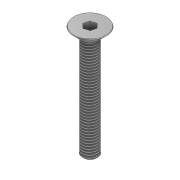
# Autodesk Inventor part: Tornillo Allen cabeza fresada M3x20mm
Saved by Autodesk Inventor 2020.3 (Build 243373000, 373)
## iProperties
Created: 2020-05-08
Part Number: Tornillo Allen cabeza fresada M3x20mm
Material: Generic
Document SubType Name: Modeling
Designer: Dante
Density: 1 g/cm^3
Appearance: Rubber - Black - Version 1.1
Mass: 0.242439 g
Surface Area: 2.80465 cm^2
Volume: 0.242439 cm^3
Author: Dante
Autodesk Inventor part; units mm, degrees
ref_plane "YZ Plane" through (0, 0, 0) normal (1, 0, 0) x (0, 1, 0)
ref_plane "XZ Plane" through (0, 0, 0) normal (0, 1, 0) x (-1, 0, 0)
ref_plane "XY Plane" through (0, 0, 0) normal (0, 0, 1) x (1, 0, 0)
sketch "Sketch1" plane through (0, 0, 0) normal (0, 0, 1) x (1, 0, 0)
  line L0 (-13.7828, -22.52) -> (-10.4228, -22.52)
  line L1 (-10.4228, -22.52) -> (-10.4228, -29.38)
  line L2 (-10.4228, -29.38) -> (-10.4228, -44.38)
  line L3 (-10.4228, -44.38) -> (-11.9228, -44.38)
  line L4 (-11.9228, -44.38) -> (-11.9228, -24.38)
  line L5 (-11.9228, -24.38) -> (-13.7828, -22.52)
  point P0 (0, 0)
  dimension "d3" = 1.5
  dimension "d15" = 1.86
  dimension "d16" = 3.36
  dimension "d23" = 20
  dimension "d24" = 21.86
  constraints: 12 end point, 2 perpendicular, 2 vertical
  measures "d3" distance of L2.end L3.end
  measures "d15" distance from line of L0 L4.end
  measures "d16" distance of L0.end L0.start
  measures "d23" distance of L3.end L4.end
  measures "d24" distance from line of L2.end L0
revolve "Revolution1" add sketch "Sketch1" angle 360 about axis through (-10.4228, -29.38, 0) along (0, -1, 0)
chamfer "Chamfer2" distance 0.2 angle 45 1 edges at (-8.9228, -44.38, 0)
chamfer "Chaflán3" distance 0.2 angle 45 1 edges at (-7.0628, -22.52, 0)
sketch "Boceto2" plane through (-10.4228, -22.52, 0) normal (0, 1, 0) x (1, 0, 0)
  line L0 (-0.8371, 0.7954) -> (0.2703, 1.1226)
  line L1 (0.2703, 1.1226) -> (1.1074, 0.3272)
  line L2 (1.1074, 0.3272) -> (0.8371, -0.7954)
  line L3 (0.8371, -0.7954) -> (-0.2703, -1.1226)
  line L4 (-0.2703, -1.1226) -> (-1.1074, -0.3272)
  line L5 (-1.1074, -0.3272) -> (-0.8371, 0.7954)
  point P0 (10.4228, 0)
  point P1 (0, 0)
  dimension "d20" = 2
  constraints: 12 end point, 13 other
  measures "d20" distance between parallel lines of L1 L4
extrude "Extrusión1" cut sketch "Boceto2" against normal blind 1.5
thread "Thread2" size "M3x0.5" class "6g" standard "ISO Metric profile" length 98
body "Solid1"
